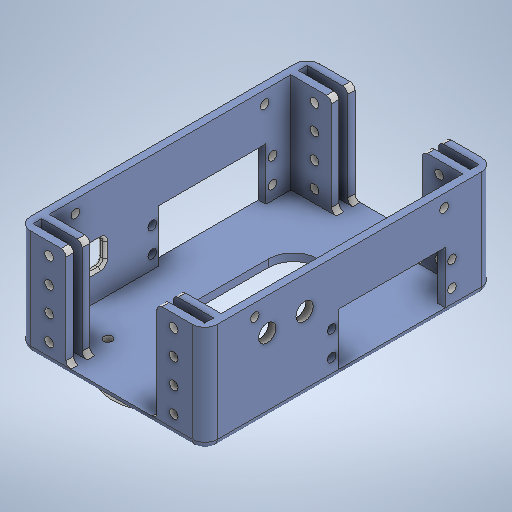
# Autodesk Inventor part: chassis
Saved by Autodesk Inventor 2025 (Build 290162000, 162)
## iProperties
Created: 2024-09-04
Part Number: chassis
Material: Générique
Document SubType Name: Modeling
Designer: chass
Density: 1 g/cm^3
Appearance: Par défaut
Author: chass
## iProperties of the stored document chassis_Impression 3D.ipt
Created: 2024-09-05
Part Number: chassis_Impression 3D
Material: Générique
Document SubType Name: Modeling
Designer: chass
Density: 1 g/cm^3
Appearance: Par défaut
Author: chass
Autodesk Inventor part; units mm, degrees
ref_plane "YZ Plane" through (0, 0, 0) normal (1, 0, 0) x (0, 1, 0)
ref_plane "XZ Plane" through (0, 0, 0) normal (0, 1, 0) x (-1, 0, 0)
ref_plane "XY Plane" through (0, 0, 0) normal (0, 0, 1) x (1, 0, 0)
sketch "Esquisse1" plane through (0, 0, 0) normal (0, 1, 0) x (-1, 0, 0)
  line L0 (37.5, 58) -> (-37.5, 58)
  line L1 (-37.5, 58) -> (-37.5, -58)
  line L2 (-37.5, -58) -> (37.5, -58)
  line L3 (37.5, -58) -> (37.5, 58)
  line L4 (37.5, 58) -> (-37.5, -58)
  line L5 (-37.5, 58) -> (37.5, -58)
  point P0 (0, 0)
  point P1 (0, 0)
  point P2 (0, 0)
  dimension "d73" = 75
  dimension "d74" = 116
  constraints: 12 end point, 2 midpoint, 2 parallel, 1 coincident, 1 horizontal, 1 perpendicular
  measures "d73" distance of L1.end L2.end
  measures "d74" distance of L0.end L1.end
extrude "Extrusion1" add sketch "Esquisse1" along normal blind 3
sketch "Esquisse2" plane through (0, 3, 0) normal (0, 1, 0) x (1, 0, 0)
  line L0 (-37.5, 58) -> (-37.5, -58) projected
  line L1 (37.5, 58) -> (-37.5, 58) projected
  line L2 (-37.5, -58) -> (-34.5, -58)
  line L3 (-34.5, -58) -> (-34.5, 58)
  line L4 (-34.5, 58) -> (-37.5, 58)
  line L5 (-37.5, 58) -> (-37.5, -58)
  line L6 (0, -93.4559) -> (0, 106.1011)
  line L7 (37.5, 58) -> (37.5, -58)
  line L8 (-37.5, 58) -> (37.5, 58)
  line L9 (37.5, -58) -> (34.5, -58)
  line L10 (34.5, -58) -> (34.5, 58)
  line L11 (-34.5, -58) -> (-18.25, -58)
  line L12 (-18.25, -58) -> (-18.25, -55)
  line L13 (-18.25, -55) -> (-34.5, -55)
  line L14 (-34.5, -55) -> (-34.5, -58)
  line L15 (-34.5, -51.5) -> (-18.25, -51.5)
  line L16 (-18.25, -51.5) -> (-18.25, -48.5)
  line L17 (-18.25, -48.5) -> (-34.5, -48.5)
  line L18 (-34.5, -48.5) -> (-34.5, -51.5)
  line L19 (-63.4161, 0) -> (50.7812, 0)
  line L20 (34.5, -58) -> (18.25, -58)
  line L21 (18.25, -58) -> (18.25, -55)
  line L22 (18.25, -55) -> (34.5, -55)
  line L23 (34.5, -55) -> (34.5, -58)
  line L24 (34.5, -51.5) -> (18.25, -51.5)
  line L25 (18.25, -51.5) -> (18.25, -48.5)
  line L26 (18.25, -48.5) -> (34.5, -48.5)
  line L27 (34.5, -48.5) -> (34.5, -51.5)
  line L28 (63.4161, 0) -> (-50.7812, 0)
  line L29 (-34.5, 58) -> (-18.25, 58)
  line L30 (-18.25, 58) -> (-18.25, 55)
  line L31 (-18.25, 55) -> (-34.5, 55)
  line L32 (-34.5, 55) -> (-34.5, 58)
  line L33 (-34.5, 51.5) -> (-18.25, 51.5)
  line L34 (-18.25, 51.5) -> (-18.25, 48.5)
  line L35 (-18.25, 48.5) -> (-34.5, 48.5)
  line L36 (-34.5, 48.5) -> (-34.5, 51.5)
  line L37 (18.25, 51.5) -> (18.25, 48.5)
  line L38 (18.25, 48.5) -> (34.5, 48.5)
  line L39 (18.25, 55) -> (34.5, 55)
  line L40 (18.25, 58) -> (18.25, 55)
  line L41 (34.5, 58) -> (18.25, 58)
  line L42 (34.5, 55) -> (34.5, 58)
  line L43 (34.5, 48.5) -> (34.5, 51.5)
  line L44 (34.5, 51.5) -> (18.25, 51.5)
  line L45 (37.5, -58) -> (37.5, 58) projected
  point P0 (0, 0)
  point P1 (34.5, 58)
  point P2 (-26.375, -55)
  point P3 (-26.375, -51.5)
  point P4 (26.375, -55)
  point P5 (26.375, -51.5)
  point P6 (-26.375, 55)
  point P7 (-26.375, 51.5)
  point P8 (26.375, 55)
  point P9 (26.375, 51.5)
  point P10 (34.5, 48.5)
  point P11 (34.5, 51.5)
  point P12 (34.5, 55)
  point P13 (18.25, 58)
  point P14 (-34.5, 51.5)
  point P15 (-34.5, 48.5)
  point P16 (-34.5, 55)
  point P17 (-18.25, 58)
  dimension "d2" = 3
  dimension "d6" = 3
  dimension "d8" = 3
  dimension "d112" = 18.25
  dimension "d113" = 3.5
  constraints: 86 end point, 34 symmetric about line, 6 parallel, 4 horizontal, 3 perpendicular, 3 point on line, 2 midpoint, 1 collinear, 1 vertical
  measures "d2" distance of L4.end L3.end
  measures "d6" distance of L12.end L11.end
  measures "d8" distance of L15.end L16.end
  measures "d112" distance between parallel lines of L6 L12
  measures "d113" distance between parallel lines of L15 L13
extrude "Extrusion2" add sketch "Esquisse2" along normal blind 40 contours L1 L3 L19 L0 | L19 L3 L2 L0 | L1 L30 L31 L3 | L3 L13 L12 L11 | L17 L16 L15 L3 | L3 L33 L34 L35 | L19 L7 L9 L10 | L10 L1 L7 L19 | L1 L10 L39 L40 | L10 L24 L25 L26 | L38 L37 L44 L10 | L10 L20 L21 L22
sketch "Esquisse3" plane through (37.5, 0, 58) normal (1, 0, 0) x (0, 0, -1)
  line L0 (0, 0) -> (116, 0) projected
  line L1 (116, 0) -> (116, 43) projected
  line L2 (0, 3) -> (0, 43) projected
  line L3 (9.5, 43) -> (106.5, 43) projected
  line L4 (53.5, 24) -> (96.5, 24)
  line L5 (96.5, 24) -> (96.5, 3)
  line L6 (96.5, 3) -> (53.5, 3)
  line L7 (53.5, 3) -> (53.5, 24)
  line L8 (0, 43) -> (116, 0)
  line L9 (116, 43) -> (0, 0)
  circle A0 centre (50.85, 18.5) radius 1.75
  circle A1 centre (50.86, 8.5) radius 1.75
  line L10 (53.5, 13.5) -> (96.5, 13.5)
  line L11 (75, 3) -> (75, 24)
  circle A2 centre (99.15, 18.5) radius 1.75
  circle A3 centre (99.14, 8.5) radius 1.75
  circle A4 centre (20, 38) radius 1.75
  line L12 (9.5, 3) -> (9.5, 43) projected
  circle A5 centre (96, 38) radius 1.75
  point P0 (58, 0)
  point P1 (50, 21.5)
  point P2 (58, 21.5)
  point P3 (58, 21.5)
  dimension "d54" = 43
  dimension "d55" = 21
  dimension "d97" = 3.5
  dimension "d123" = 3
  dimension "d124" = 5
  dimension "d125" = 10
  dimension "d127" = 75
  dimension "d128" = 24.15
  dimension "d129" = 24.14
  dimension "d139" = 3.5
  dimension "d141" = 20
  dimension "d142" = 5
  dimension "d143" = 3.5
  dimension "d144" = 20
  dimension "d145" = 5
  constraints: 16 end point, 6 centre point, 6 midpoint, 2 parallel, 2 symmetric about line, 1 horizontal, 1 perpendicular, 2 other
  measures "d54" distance of L5.end L6.end
  measures "d55" distance of L4.end L5.end
  measures "d97" diameter of A0
  measures "d123" distance between parallel lines of L0 L6
  measures "d124" distance from line of L10 A0.centre
  measures "d125" distance of A1.centre A0.centre
  measures "d127" distance between parallel lines of L2 L11
  measures "d128" distance from line of L11 A0.centre
  measures "d129" distance from line of L11 A1.centre
  measures "d139" diameter of A4
  measures "d141" distance from line of A4.centre L2
  measures "d142" distance from line of L3 A4.centre
  measures "d143" diameter of A5
  measures "d144" distance from line of L1 A5.centre
  measures "d145" distance from line of L3 A5.centre
extrude "Extrusion3" cut sketch "Esquisse3" against normal blind 100 contours L8 L10 L5 | L5 L6 L11 L10 L8 | A0 L9 | L9 A0 | L9 L8 L7 L4 | L4 L11 L8 L9 | L10 L8 L11 L4 L5 | L10 L11 L8 | L8 L9 L7 | L8 L11 L10 L7 L9 | L6 L7 L10 L11 | A1 | A2 | A3 | A4 | A5
fillet "Congé1" radius 5 4 edges at (37.5, 21.5, 58) (-37.5, 21.5, 58) (37.5, 21.5, -58) (-37.5, 21.5, -58)
fillet "Congé2" radius 3 8 edges at (-36.0355, 0, 56.5355) (0, 0, 58) (36.0355, 0, 56.5355) (37.5, 0, 0) (36.0355, 0, -56.5355) (0, 0, -58) (-36.0355, 0, -56.5355) (-37.5, 0, 0)
sketch "Esquisse5" plane through (0, 3, 0) normal (0, 1, 0) x (1, 0, 0)
  line L0 (-15, -30) -> (15, -30)
  line L1 (15, -30) -> (15, 30)
  line L2 (15, 30) -> (-15, 30)
  line L3 (-15, 30) -> (-15, -30)
  line L4 (-15, -30) -> (15, 30)
  line L5 (15, -30) -> (-15, 30)
  point P0 (0, 0)
  point P1 (0, 0)
  point P2 (0, 0)
  dimension "d106" = 60
  dimension "d107" = 30
  constraints: 12 end point, 2 midpoint, 2 parallel, 1 coincident, 1 horizontal, 1 perpendicular
  measures "d106" distance of L2.end L0.start
  measures "d107" distance of L1.end L2.end
extrude "Extrusion5" cut sketch "Esquisse5" against normal blind 3
fillet "Congé5" radius 10 4 edges at (-15, 1.5, 30) (-15, 1.5, -30) (15, 1.5, 30) (15, 1.5, -30)
sketch "Esquisse6" plane through (-32.5, 43, 58) normal (0, 0, 1) x (1, 0, 0)
  circle A0 centre (7.5, -14.9609) radius 1.75
  line L0 (-5, 0) -> (-5, -40) projected
  line L1 (-5, 0) -> (70, 0)
  line L2 (70, 0) -> (70, -43)
  line L3 (70, -43) -> (-5, -43)
  line L4 (-5, -43) -> (-5, 0)
  line L5 (-5, -19.9609) -> (70, -19.9609)
  line L6 (32.5, -43) -> (32.5, 0)
  circle A1 centre (7.5, -4.9609) radius 1.75
  circle A2 centre (7.5, -24.9609) radius 1.75
  circle A3 centre (7.5, -34.9609) radius 1.75
  circle A4 centre (57.5, -14.9609) radius 1.75
  circle A5 centre (57.5, -4.9609) radius 1.75
  circle A6 centre (57.5, -24.9609) radius 1.75
  circle A7 centre (57.5, -34.9609) radius 1.75
  dimension "d114" = 3.5
  dimension "d115" = 5
  dimension "d116" = 25
  dimension "d117" = 3.5
  dimension "d118" = 10
  constraints: 12 end point, 8 centre point, 6 symmetric about line, 2 parallel, 2 perpendicular, 2 point on line, 1 horizontal, 1 midpoint, 6 other
  measures "d114" diameter of A0
  measures "d115" distance from line of L5 A0.centre
  measures "d116" distance from line of A0.centre L6
  measures "d117" diameter of A1
  measures "d118" distance of A0.centre A1.centre
extrude "Extrusion6" cut sketch "Esquisse6" against normal blind 143.25 contours A0 | A1 | A2 | A3 | A4 | A5 | A6 | A7
fillet "Congé6" radius 2 8 edges at (-18.25, 3, 50) (-18.25, 3, 56.5) (18.25, 3, 56.5) (18.25, 3, 50) (18.25, 3, -50) (18.25, 3, -56.5) (-18.25, 3, -56.5) (-18.25, 3, -50)
fillet "Congé7" radius 2 8 edges at (-18.25, 43, -56.5) (-18.25, 43, -50) (18.25, 43, -56.5) (18.25, 43, -50) (-18.25, 43, 50) (-18.25, 43, 56.5) (18.25, 43, 50) (18.25, 43, 56.5)
sketch "Esquisse7" plane through (0, 0, 0) normal (0, -1, 0) x (1, 0, 0)
  line L0 (0, 67.9334) -> (0, -81.5349)
  circle A0 centre (19.4, 40) radius 1.75
  line L1 (61.585, 0) -> (-48.9976, 0)
  circle A1 centre (-19.4, 40) radius 1.75
  point P0 (0, 0)
  dimension "d130" = 3.5
  dimension "d131" = 40
  dimension "d132" = 19.4
  dimension "d133" = 0
  constraints: 4 end point, 2 centre point, 1 horizontal, 1 point on line, 1 symmetric about line, 1 vertical, 1 other
  measures "d130" diameter of A0
  measures "d131" distance from line of L1 A0.centre
  measures "d132" distance from line of L0 A0.centre
  measures "d133" distance from line of point (0, 0) L0
extrude "Extrusion7" cut sketch "Esquisse7" against normal blind 3
sketch "Esquisse8" plane through (0, 0, 0) normal (0, -1, 0) x (1, 0, 0)
  circle A0 centre (0, 40) radius 17.5
  line L0 (13.6107, 51) -> (-9.0139, 55)
  line L1 (-32.5, 55) -> (32.5, 55) projected
  circle A1 centre (19.4, 40) radius 1.75 projected
  circle A2 centre (-19.4, 40) radius 1.75 projected
  line L2 (19.4, 40) -> (-19.4, 40)
  point P0 (0, 0)
  point P1 (32.5, 55)
  dimension "d136" = 35
  constraints: 4 end point, 2 point on circle, 1 centre point, 1 horizontal, 1 midpoint, 2 other
  measures "d136" diameter of A0
extrude "Extrusion8" add sketch "Esquisse8" against normal blind 3 contours L0 L1 A0 | L1 A0
sketch "Esquisse9" plane through (-37.5, 24, -38.5) normal (-1, 0, 0) x (0, 0, 1)
  line L0 (64.5, 0) -> (79.5, 0)
  line L1 (79.5, 0) -> (79.5, -10)
  line L2 (79.5, -10) -> (64.5, -10)
  line L3 (64.5, -10) -> (64.5, 0)
  line L4 (91.5, -21) -> (43, -21) projected
  line L5 (64.5, 0) -> (79.5, -10)
  line L6 (64.5, -10) -> (79.5, 0)
  line L7 (96.5, -21) -> (96.5, 19) projected
  line L8 (87, -21) -> (87, 19) projected
  point P0 (38.5, -24)
  point P1 (72, -5)
  point P2 (72, -5)
  dimension "d146" = 15
  dimension "d147" = 10
  dimension "d149" = 16
  dimension "d164" = 15
  constraints: 12 end point, 2 midpoint, 2 parallel, 1 horizontal, 1 perpendicular
  measures "d146" distance of L1.end L2.end
  measures "d147" distance of L0.end L1.end
  measures "d149" distance from line of L4 point (72, -5)
  measures "d164" distance from line of L8 point (72, -5)
extrude "Extrusion9" cut sketch "Esquisse9" against normal blind 3
fillet "Congé8" radius 2 4 edges at (-36, 24, 26) (-36, 14, 26) (-36, 14, 41) (-36, 24, 41)
fillet "Congé9" radius 1 16 edges at (-37.5, 14, 33.5) (-37.5, 14.5858, 26.5858) (-37.5, 19, 26) (-37.5, 23.4142, 26.5858) (-37.5, 24, 33.5) (-37.5, 23.4142, 40.4142) (-37.5, 19, 41) (-37.5, 14.5858, 40.4142) (-34.5, 19, 26) (-34.5, 23.4142, 26.5858) (-34.5, 24, 33.5) (-34.5, 23.4142, 40.4142) (-34.5, 19, 41) (-34.5, 14.5858, 40.4142) (-34.5, 14, 33.5) (-34.5, 14.5858, 26.5858)
sketch "Esquisse10" plane through (37.5, 24, 4.5) normal (1, 0, 0) x (0, 0, -1)
  circle A0 centre (-13.5, 6) radius 3.5
  line L0 (0, -21) -> (-48.5, -21) projected
  circle A1 centre (-28.5, 6) radius 3.5
  line L1 (-53.5, 19) -> (-53.5, -21) projected
  point P0 (4.5, -24)
  dimension "d154" = 7
  dimension "d155" = 27
  dimension "d158" = 7
  dimension "d159" = 15
  dimension "d160" = 25
  dimension "d161" = 27
  constraints: 2 centre point
  measures "d154" diameter of A0
  measures "d155" distance from line of L0 A0.centre
  measures "d158" diameter of A1
  measures "d159" distance of A0.centre A1.centre
  measures "d160" distance from line of A1.centre L1
  measures "d161" distance from line of A1.centre L0
extrude "Extrusion10" cut sketch "Esquisse10" against normal blind 3
